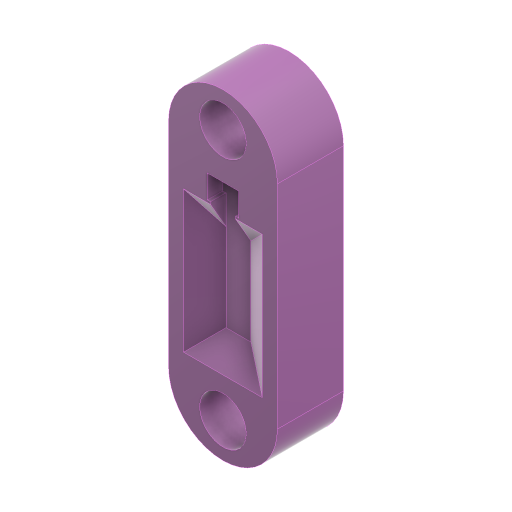
# Autodesk Inventor part: Установка датчика холла
Saved by Autodesk Inventor 2024.1 (Build 281209000, 209)
## iProperties
Created: 2023-03-30
Part Number: Установка датчика холла
Material: Типовые
Document SubType Name: Modeling
Designer: Admin
Density: 1 g/cm^3
Appearance: По умолчанию
Author: Admin
Autodesk Inventor part; units mm, degrees
ref_plane "YZ Plane" through (0, 0, 0) normal (1, 0, 0) x (0, 1, 0)
ref_plane "XZ Plane" through (0, 0, 0) normal (0, 1, 0) x (-1, 0, 0)
ref_plane "XY Plane" through (0, 0, 0) normal (0, 0, 1) x (1, 0, 0)
sketch "Эскиз1" plane through (0, 0, 0) normal (0, 0, 1) x (1, 0, 0)
  line L0 (-2.03, 1.5) -> (2.03, 1.5)
  line L1 (2.03, 1.5) -> (2.03, -1.5)
  line L2 (2.03, -1.5) -> (-2.03, -1.5)
  line L3 (-2.03, -1.5) -> (-2.03, 1.5)
  line L4 (-2.03, 1.5) -> (2.03, -1.5) construction
  line L5 (2.03, 1.5) -> (-2.03, -1.5) construction
  line L6 (-1.6, -1.5) -> (1.6, -1.5)
  line L7 (1.6, -1.5) -> (1.6, -16.5)
  line L8 (1.6, -16.5) -> (-1.6, -16.5)
  line L9 (-1.6, -16.5) -> (-1.6, -1.5)
  line L10 (0, 4.8) -> (0, -22.5041) construction
  line L11 (-7, 4.8) -> (-7, -22.5041)
  line L12 (7, -22.5041) -> (7, 4.8)
  arc A0 (7, 4.8) -> (-7, 4.8) centre (0, 4.8) ccw
  arc A1 (-7, -22.5041) -> (7, -22.5041) centre (0, -22.5041) ccw
  line L13 (-1.6, -1.5) -> (-1.6, -9)
  line L14 (1.6, -1.5) -> (1.6, -9)
  line L15 (-1.6, -5.25) -> (-5.6947, -16.5)
  line L16 (1.6, -5.25) -> (5.6947, -16.5)
  arc A2 (-5.6947, -16.5) -> (5.6947, -16.5) centre (0, -0.854) ccw
  line L17 (1.6, -5.25) -> (-1.6, -5.25)
  circle A3 centre (0, -25.0041) radius 1.5
  circle A4 centre (0, 7.3) radius 1.5
  point P0 (0, 0)
  point P1 (0, 0)
  point P2 (0, 0)
  point P3 (0, 0)
  point P4 (0, -1.5)
  point P5 (0, 0)
  point P6 (0, -8.8521)
  point P7 (1.6, -5.25)
  point P8 (-1.6, -5.25)
  point P9 (1.6, -1.5)
  dimension "d0" = 4.06
  dimension "d1" = 3
  dimension "d2" = 3.2
  dimension "d3" = 15
  dimension "d4" = 14
  dimension "d5" = 20
  dimension "d6" = 20
  dimension "d15" = 3
  dimension "d16" = 3
  dimension "d17" = 3
  dimension "d18" = 3
  dimension "d20" = 6
  dimension "d24" = 16.1521
  constraints: 38 end point, 8 midpoint, 6 point on circle, 5 centre point, 5 parallel, 4 coincident, 4 tangent, 4 vertical alignment, 3 horizontal, 2 line through centre, 2 perpendicular, 1 horizontal alignment, 1 point on line, 1 vertical
  measures "d0" distance of L3.end L0.end
  measures "d1" distance of L0.end L2.start
  measures "d2" distance of L7.end L9.start
  measures "d3" distance of L7.start L7.end
  measures "d4" diameter of A1
  measures "d5" angle of L7 L16
  measures "d6" angle of L9 L15
  measures "d15" diameter of A3
  measures "d16" diameter of A4
  measures "d24" distance of point (0, -8.852) A4.centre
extrude "Выдавливание1" add sketch "Эскиз1" along normal blind 2 and the other way blind 6.5 contours L0 L1 L2 L3 | L2 L7 L17 L9 | L17 L7 L8 L9 | L9 L8 L7 L16 A2 L15 | A0 L12 A1 L11
extrude "Выдавливание2" cut sketch "Эскиз1" along normal up to surface (2 mm away) draft 60 contours L17 L7 L8 L9
extrude "Выдавливание3" cut sketch "Эскиз1" along normal up to surface (2 mm away) contours L0 L1 L2 L3 | L2 L7 L17 L9
sketch "Эскиз2" plane through (0, 0, 2) normal (0, 0, 1) x (1, 0, 0)
  circle A0 centre (0, 7.3) radius 1.5 projected
  circle A1 centre (0, -25.0041) radius 1.5 projected
  circle A2 centre (0, 7.3) radius 3
  circle A3 centre (0, -25.0041) radius 3
  point P0 (0, 0)
  dimension "d21" = 6
  constraints: 2 centre point, 2 coincident, 1 equal radius
  measures "d21" diameter of A2
extrude "Выдавливание4" cut sketch "Эскиз2" against normal blind 5.5 contours A0 | A1 | A2 | A3
